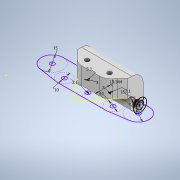
# Autodesk Inventor part: prig to kauri conversion front link
Saved by Autodesk Inventor 2020 (Build 240168000, 168)
## iProperties
Created: 2022-05-24
Part Number: prig to kauri conversion front link
Material: Generic
Document SubType Name: Modeling
Designer: Steven
Density: 1 g/cm^3
Appearance: Default
Author: Steven
Autodesk Inventor part; units mm, degrees
ref_plane "YZ Plane" through (0, 0, 0) normal (1, 0, 0) x (0, 1, 0)
ref_plane "XZ Plane" through (0, 0, 0) normal (0, 1, 0) x (-1, 0, 0)
ref_plane "XY Plane" through (0, 0, 0) normal (0, 0, 1) x (1, 0, 0)
sketch "Sketch1" plane through (0, 0, 0) normal (0, 1, 0) x (-1, 0, 0)
  circle A0 centre (-30, -5.1319) radius 1.5
  arc A1 (-31.1155, 2.2846) -> (-30, -12.6319) centre (-30, -5.1319) ccw
  arc A2 (-30, -12.6319) -> (-31.1155, 2.2846) centre (-30, -5.1319) ccw construction
  circle A3 centre (-16.9706, -0.5878) radius 1.5
  circle A4 centre (16.9706, -0.5878) radius 1.5
  circle A5 centre (16.9706, -0.5878) radius 5 construction
  line L0 (-16.9706, 4.4122) -> (-31.1155, 2.2846)
  circle A6 centre (-16.9706, -0.5878) radius 5 construction
  circle A7 centre (-7.8058, -8.4213) radius 1.55
  line L1 (0, -8.4213) -> (-15.6117, -8.4213) construction
  circle A8 centre (0, 0) radius 1.55
  line L2 (-16.9706, 4.4122) -> (16.9706, 4.4122)
  line L3 (30, -12.6319) -> (-30, -12.6319)
  circle A9 centre (30, -5.1319) radius 1.5
  line L4 (0, 4.2106) -> (0, -4.2106) construction
  line L5 (0, -4.2106) -> (0, -12.6319) construction
  line L6 (0, -4.2106) -> (3.1574, -4.2106) construction
  line L7 (0, -8.4213) -> (15.6117, -8.4213) construction
  line L8 (16.9706, 4.4122) -> (31.1155, 2.2846)
  arc A10 (31.1155, 2.2846) -> (30, -12.6319) centre (30, -5.1319) ccw construction
  arc A11 (30, -12.6319) -> (31.1155, 2.2846) centre (30, -5.1319) ccw
  circle A12 centre (7.8058, -8.4213) radius 1.55
  point P0 (0, 0)
  point P1 (0, 0)
  dimension "d0" = 10
  dimension "d1" = 10
  dimension "d2" = 15
  dimension "d3" = 15
  dimension "d4" = 3.1
  dimension "d5" = 3.1
  dimension "d6" = 3.1
  constraints: 18 end point, 11 centre point, 8 point on circle, 5 midpoint, 4 coincident, 4 horizontal, 3 tangent, 2 vertical alignment, 1 point on line, 4 other
  measures "d2" diameter of A1
  measures "d3" diameter of A11
  measures "d4" diameter of A8
  measures "d5" diameter of A12
  measures "d6" diameter of A7
sketch "Sketch2" plane through (0, 0, 0) normal (0, 1, 0) x (-1, 0, 0)
  circle A0 centre (15, 9.8681) radius 3
  circle A1 centre (16.9706, -0.5878) radius 1.5
  arc A2 (3.1574, 6.6664) -> (-3.1574, 6.6664) centre (0, 4.2106) ccw
  line L0 (3.1574, 6.6664) -> (11.0366, -3.464)
  arc A3 (11.0366, -3.464) -> (13.9152, -6.7248) centre (38.6639, 18.024) ccw
  line L1 (13.9152, -6.7248) -> (21.1612, -13.9708)
  arc A4 (30.0072, 37.5736) -> (30.286, 34.6489) centre (32.7505, 36.3595) ccw
  arc A5 (35.8309, 43.8114) -> (30.0072, 37.5736) centre (41.895, 32.3124) ccw
  circle A6 centre (25.4558, 41.8386) radius 1.5
  circle A7 centre (30, 54.8681) radius 1.5
  circle A8 centre (16.9706, 50.3239) radius 1.5
  circle A9 centre (15, 39.8681) radius 3
  circle A10 centre (24.2029, 72.4055) radius 1.5
  line L2 (27.7949, 74.3102) -> (17.0958, 107.9924)
  arc A11 (17.0958, 107.9924) -> (14.6505, 110.5406) centre (13.2835, 106.7814) ccw
  circle A12 centre (13.2835, 106.7814) radius 1.5
  line L3 (14.6505, 110.5406) -> (2.0505, 115.1224)
  circle A13 centre (-24.2029, 72.4055) radius 1.5
  arc A14 (2.0505, 115.1224) -> (-2.0505, 115.1224) centre (0, 109.4837) ccw
  line L4 (-17.0958, 107.9924) -> (-27.7949, 74.3102)
  circle A15 centre (-13.2835, 106.7814) radius 1.5
  arc A16 (-14.6505, 110.5406) -> (-17.0958, 107.9924) centre (-13.2835, 106.7814) ccw
  line L5 (-2.0505, 115.1224) -> (-14.6505, 110.5406)
  line L6 (-25.5, 17.3681) -> (-25.5, 32.3681)
  line L7 (-28.5, 32.3681) -> (-28.5, 17.3681)
  line L8 (-31, 32.3681) -> (-31, 17.3681)
  arc A17 (-28.5, 17.3681) -> (-25.5, 17.3681) centre (-27, 17.3681) ccw
  arc A18 (-31, 17.3681) -> (-30.286, 15.0873) centre (-27, 17.3681) ccw
  arc A19 (-30.0072, 37.5736) -> (-35.8309, 43.8114) centre (-41.895, 32.3124) ccw
  arc A20 (-25.5, 32.3681) -> (-28.5, 32.3681) centre (-27, 32.3681) ccw
  arc A21 (-30.286, 34.6489) -> (-31, 32.3681) centre (-27, 32.3681) ccw
  arc A22 (-30.286, 34.6489) -> (-30.0072, 37.5736) centre (-32.7505, 36.3595) ccw
  circle A23 centre (-25.4558, 41.8386) radius 1.5
  circle A24 centre (-15, 39.8681) radius 3
  circle A25 centre (-16.9706, 50.3239) radius 1.5
  arc A26 (-30.0072, 12.1625) -> (-30.286, 15.0873) centre (-32.7505, 13.3766) ccw
  arc A27 (-35.8309, 5.9248) -> (-30.0072, 12.1625) centre (-41.895, 17.4238) ccw
  arc A28 (-35.8309, 5.9248) -> (-21.1612, -13.9708) centre (-30, -5.1319) ccw
  line L9 (-21.1612, -13.9708) -> (-13.9152, -6.7248)
  circle A29 centre (-15, 9.8681) radius 3
  circle A30 centre (-25.4558, 7.8975) radius 1.5
  circle A31 centre (-16.9706, -0.5878) radius 1.5
  circle A32 centre (-30, -5.1319) radius 1.5
  line L10 (-11.0366, -3.464) -> (-3.1574, 6.6664)
  arc A33 (-13.9152, -6.7248) -> (-11.0366, -3.464) centre (-38.6639, 18.024) ccw
  line L11 (31, 17.3681) -> (31, 32.3681)
  arc A34 (28.5, 32.3681) -> (25.5, 32.3681) centre (27, 32.3681) ccw
  line L12 (25.5, 32.3681) -> (25.5, 17.3681)
  line L13 (28.5, 17.3681) -> (28.5, 32.3681)
  arc A35 (31, 32.3681) -> (30.286, 34.6489) centre (27, 32.3681) ccw
  arc A36 (-34.9925, 66.3278) -> (-27.7949, 74.3102) centre (-40.1848, 78.2458) ccw
  arc A37 (-34.9925, 66.3278) -> (-35.8309, 43.8114) centre (-30, 54.8681) ccw
  circle A38 centre (-30, 54.8681) radius 1.5
  arc A39 (30.0072, 12.1625) -> (35.8309, 5.9248) centre (41.895, 17.4238) ccw
  circle A40 centre (30, -5.1319) radius 1.5
  arc A41 (21.1612, -13.9708) -> (35.8309, 5.9248) centre (30, -5.1319) ccw
  circle A42 centre (25.4558, 7.8975) radius 1.5
  arc A43 (25.5, 17.3681) -> (28.5, 17.3681) centre (27, 17.3681) ccw
  arc A44 (30.286, 15.0873) -> (30.0072, 12.1625) centre (32.7505, 13.3766) ccw
  arc A45 (30.286, 15.0873) -> (31, 17.3681) centre (27, 17.3681) ccw
  arc A46 (35.8309, 43.8114) -> (34.9925, 66.3278) centre (30, 54.8681) ccw
  arc A47 (27.7949, 74.3102) -> (34.9925, 66.3278) centre (40.1848, 78.2458) ccw
  circle A48 centre (-30, -5.1319) radius 1.5 construction
  point P0 (0, 0)
  point P1 (0, 109.4837)
  constraints: 56 point on circle, 48 centre point, 28 end point
sketch "Sketch3" plane through (0, 0, 0) normal (0, 1, 0) x (-1, 0, 0)
  arc A0 (3.1574, 6.6664) -> (-3.1574, 6.6664) centre (0, 4.2106) ccw projected
  line L0 (-11.0366, -3.464) -> (-3.1574, 6.6664) projected
  line L1 (3.1574, 6.6664) -> (11.0366, -3.464) projected
  arc A1 (11.0366, -3.464) -> (13.9152, -6.7248) centre (38.6639, 18.024) ccw projected
  arc A2 (-13.9152, -6.7248) -> (-11.0366, -3.464) centre (-38.6639, 18.024) ccw projected
  line L2 (-21.1612, -13.9708) -> (-13.9152, -6.7248) projected
  line L3 (13.9152, -6.7248) -> (21.1612, -13.9708) projected
  line L4 (30, -12.6319) -> (-30, -12.6319) projected
  circle A3 centre (-7.8058, -8.4213) radius 1.55 construction
  circle A4 centre (7.8058, -8.4213) radius 1.55 construction
  circle A5 centre (0, 0) radius 1.55 projected
  circle A6 centre (-16.9706, -0.5878) radius 1.5 construction
  circle A7 centre (16.9706, -0.5878) radius 1.5 construction
  line L5 (-16.9706, -2.0878) -> (16.9706, -2.0878) construction
  line L6 (7.8058, -12.6319) -> (7.8058, -2.0878) construction
  line L7 (-7.8058, -12.6319) -> (-7.8058, -2.0878) construction
  circle A8 centre (-7.8058, -7.3599) radius 1.5
  circle A9 centre (7.8058, -7.3599) radius 1.5
  line L8 (-5.032, -12.6319) -> (-5.032, -2.0878) construction
  line L9 (-5.032, -7.3599) -> (-10.6888, -7.3599) construction
  point P0 (0, 0)
  point P1 (-19.8223, -12.6319)
  point P2 (19.8223, -12.6319)
  dimension "d38" = 3
  dimension "d39" = 3
  dimension "d42" = 10.5442
  constraints: 10 end point, 6 point on line, 3 perpendicular, 2 centre point, 2 horizontal, 2 vertical alignment, 1 midpoint, 2 other
  measures "d38" diameter of A8
  measures "d39" diameter of A9
  measures "d42" distance of L8.start L8.end
extrude "Extrusion1" add sketch "Sketch3" along normal blind 6 contours L1 A1 L3 L4 L2 A2 L0 A0 | A8 | A9
sketch "Sketch4" plane through (19.8223, 0, -12.6319) normal (0, 0, -1) x (-1, 0, 0)
  line L0 (0, 0) -> (39.6447, 0) projected
  line L1 (39.6447, 0) -> (39.6447, 6) projected
  line L2 (0, 6) -> (39.6447, 6) projected
  line L3 (0, 0) -> (0, 6) projected
  point P0 (19.8223, 0)
extrude "Extrusion2" add sketch "Sketch4" along normal blind 8.5
sketch "Sketch5" plane through (0, 0, 0) normal (0, -1, 0) x (1, 0, 0)
  line L0 (-19.8223, -21.1319) -> (19.8223, -21.1319) projected
  line L1 (19.8223, -21.1319) -> (19.8223, -13.6319)
  line L2 (19.8223, -12.6319) -> (19.8223, -21.1319) projected
  line L3 (19.8223, -13.6319) -> (-19.8223, -13.6319)
  line L4 (-19.8223, -12.6319) -> (-19.8223, -21.1319) projected
  line L5 (-19.8223, -13.6319) -> (-19.8223, -21.1319)
  line L6 (-19.8223, -21.1319) -> (19.8223, -21.1319)
  point P0 (0, 0)
  dimension "d11" = 7.5
  constraints: 8 end point, 2 perpendicular, 2 point on line, 1 vertical
  measures "d11" distance of L0.end L1.end
extrude "Extrusion3" add sketch "Sketch5" along normal blind 7
sketch "Sketch6" plane through (19.8223, 6, -12.6319) normal (1, 0, 0) x (0, 0, -1)
  line L0 (0, -6) -> (0, 0) construction
  line L1 (0, -6) -> (0, -11.9599) construction
  line L2 (0, -11.9599) -> (3.918, -11.9599) construction
  circle A0 centre (3.918, -11.9599) radius 2.55
  circle A1 centre (3.918, -11.9599) radius 4.5
  line L3 (1, -6) -> (1, -13) construction
  line L4 (1, -6) -> (1, -7) construction
  line L5 (1, -7) -> (-0.2839, -10.3492)
  line L6 (1, -7) -> (1, -8.5343)
  line L7 (1, -6) -> (1, -13) projected
  point P0 (-12.6319, -6)
  dimension "d15" = 5.96
  dimension "d16" = 3.918
  dimension "d17" = 5.1
  dimension "d18" = 9
  dimension "d20" = 1
  constraints: 10 end point, 2 centre point, 2 coincident, 2 point on circle, 2 point on line, 1 perpendicular, 1 tangent, 1 vertical
  measures "d15" distance of L0.start L1.end
  measures "d16" distance of L1.end L2.end
  measures "d17" diameter of A0
  measures "d18" diameter of A1
  measures "d20" distance of L3.start L4.end
fillet "Fillet2" radius 1 1 edges at (0, 0, -13.6319)
extrude "Extrusion4" add sketch "Sketch6" against normal up to surface (39.6447 mm away) contours A1
extrude "Extrusion5" cut sketch "Sketch6" against normal up to surface (39.6447 mm away) contours A0
fillet "Fillet3" radius 3 1 edges at (0, -7, -21.1319)
extrude "Extrusion6" add sketch "Sketch6" against normal up to surface (39.6447 mm away) contours A1 L5 L6
sketch "Sketch7" plane through (0, 6, 0) normal (0, 1, 0) x (1, 0, 0)
  line L0 (-19.8223, 12.6319) -> (-13.9152, 6.7248) projected
  arc A0 (-11.0366, 3.464) -> (-13.9152, 6.7248) centre (-38.6639, -18.024) ccw projected
  line L1 (-11.0366, 3.464) -> (-3.1574, -6.6664) projected
  arc A1 (-3.1574, -6.6664) -> (3.1574, -6.6664) centre (0, -4.2106) ccw projected
  line L2 (3.1574, -6.6664) -> (11.0366, 3.464) projected
  arc A2 (13.9152, 6.7248) -> (11.0366, 3.464) centre (38.6639, -18.024) ccw projected
  line L3 (13.9152, 6.7248) -> (19.8223, 12.6319) projected
  line L4 (19.8223, 12.6319) -> (19.8223, 21.1319) projected
  line L5 (-19.8223, 21.1319) -> (19.8223, 21.1319) projected
  line L6 (-19.8223, 12.6319) -> (-19.8223, 21.1319) projected
  circle A3 centre (0, 0) radius 1.55 projected
  point P0 (0, 0)
extrude "Extrusion7" add sketch "Sketch7" along normal blind 6
fillet "Fillet4" radius 8 1 edges at (0, 12, -21.1319)
sketch "Sketch8" plane through (0, 12, 0) normal (0, 1, 0) x (1, 0, 0)
  line L0 (0, 0) -> (0, 27.291) construction
  line L1 (-0.7613, 27.291) -> (-17.5, 27.291) construction
  line L2 (0.7613, 27.291) -> (17.5, 27.291) construction
  line L3 (-17.5, 27.291) -> (-17.5, 7.1815)
  line L4 (17.5, 27.291) -> (17.5, 7.1815)
  line L5 (17.5, 7.1815) -> (23.8846, 7.1815)
  line L6 (23.8846, 7.1815) -> (23.8846, 23.5209)
  line L7 (-17.5, 7.1815) -> (-22.9652, 7.1815)
  line L8 (-22.9652, 7.1815) -> (-22.9652, 23.5209)
  line L9 (-22.9652, 23.5209) -> (23.8846, 23.5209)
  point P0 (17.5, 23.5209)
  point P1 (-17.5, 23.5209)
  dimension "d34" = 35
  constraints: 20 end point, 4 perpendicular, 3 vertical, 2 symmetric about line, 1 horizontal
  measures "d34" distance between parallel lines of L4 L3
extrude "Extrusion8" cut sketch "Sketch8" against normal through all
sketch "Sketch9" plane through (0, 0, 0) normal (0, -1, 0) x (1, 0, 0)
  circle A0 centre (0, 0) radius 1.55 projected
  circle A1 centre (-16.9706, -0.5878) radius 1.5 projected
  circle A2 centre (16.9706, -0.5878) radius 1.5 projected
  line L0 (-16.9706, -2.0878) -> (16.9706, -2.0878)
  line L1 (16.9706, -2.0878) -> (16.9706, 15.9474)
  line L2 (16.9706, 15.9474) -> (-16.9706, 15.341)
  line L3 (-16.9706, 15.341) -> (-16.9706, -2.0878)
  point P0 (0, 0)
  point P1 (-16.9706, 0.9122)
  point P2 (16.9706, 0.9122)
  constraints: 8 end point, 1 horizontal, 1 parallel, 1 vertical, 4 other
extrude "Extrusion9" cut sketch "Sketch9" against normal up to surface (12 mm away) contours A1 L3 L2 L1 A2 L0
fillet "Fillet5" radius 8 2 edges at (-9.9662, 6, -2.0878) (9.9662, 6, -2.0878)
extrude "Extrusion10" cut sketch "Sketch3" along normal up to surface (12 mm away) contours A8 | A9
body "Solid1"
